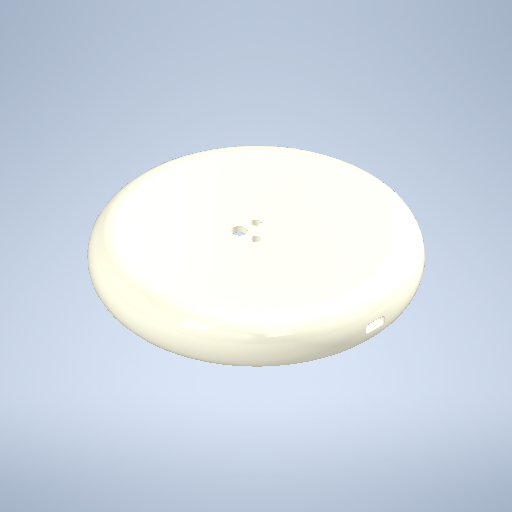
# Autodesk Inventor part: Base
Saved by Autodesk Inventor 2025.3 (Build 293356000, 356)
## iProperties
Created: 2026-01-15
Part Number: Base
Material: Acetal Resin, White
Document SubType Name: Modeling
Designer: Balint
Density: 1.425 g/cm^3
Appearance: Smooth - White
Mass: 112.917 g
Surface Area: 362.078 cm^2
Volume: 79.2398 cm^3
Author: Balint
Autodesk Inventor part; units mm, degrees
ref_plane "XZ Plane" through (0, 0, 0) normal (0, 1, 0) x (-1, 0, 0)
ref_plane "XY Plane" through (0, 0, 0) normal (0, 0, 1) x (1, 0, 0)
sketch "Sketch1" plane through (0, 0, 0) normal (0, 0, 1) x (1, 0, 0)
  line L0 (0, 0) -> (0, 22)
  line L1 (60, 5) -> (60, 5)
  line L2 (48.75, 19) -> (3, 19)
  line L3 (3, 19) -> (0, 19)
  line L4 (46.25, 0) -> (46.25, 2)
  line L5 (46.25, 2) -> (46.25, 3)
  line L6 (46.25, 3) -> (36.25, 3)
  line L7 (36.25, 3) -> (36.25, 6)
  line L8 (36.25, 6) -> (48.75, 6)
  line L9 (60, 11) -> (60, 11)
  line L10 (46.25, 0) -> (49, 0)
  line L11 (0, 22) -> (49, 22)
  arc A0 (60, 11) -> (49, 22) centre (49, 11) ccw
  arc A1 (49, 0) -> (60, 11) centre (49, 11) ccw
  line L12 (48.75, 6) -> (49.75, 6)
  line L13 (50.75, 7) -> (50.75, 18)
  line L14 (48.75, 19) -> (49.75, 19)
  arc A2 (50.75, 18) -> (49.75, 19) centre (49.75, 18) ccw
  arc A3 (49.75, 6) -> (50.75, 7) centre (49.75, 7) ccw
  point P0 (60, 22)
  point P1 (50.75, 6)
  dimension "d0" = 22
  dimension "d1" = 60
  dimension "d6" = 1
  dimension "d7" = 10
  dimension "d8" = 3
  dimension "d47" = 11
  dimension "d48" = 2
  dimension "d49" = 1
  constraints: 30 end point, 8 point on circle, 8 tangent, 6 perpendicular, 4 centre point, 3 horizontal, 3 point on line, 2 equal radius, 2 vertical
  measures "d0" distance of L0.start L0.end
  measures "d1" distance of L0.end point (60, 22)
  measures "d6" distance of L4.end L5.end
  measures "d7" distance of L5.end L6.end
  measures "d8" distance of L6.end L7.end
  measures "d47" radius of A0
  measures "d48" distance of L8.end point (50.75, 6)
  measures "d49" radius of A2
revolve "Revolution1" add sketch "Sketch1" angle 360 about axis through (0, 0, 0) along (0, 1, 0)
sketch "Sketch2" plane through (0, 3, 0) normal (0, -1, 0) x (1, 0, 0)
  circle A0 centre (0, 0) radius 36.25 projected
  circle A1 centre (0, 41.25) radius 1.9
  circle A2 centre (0, 0) radius 46.25 projected
  line L0 (0, 46.25) -> (0, 41.25)
  dimension "d11" = 3.8
  dimension "d38" = 5
  dimension "d39" = 0
  constraints: 2 end point, 1 centre point, 1 vertical, 1 vertical alignment, 1 other
  measures "d11" diameter of A1
  measures "d38" distance of L0.start L0.end
  measures "d39" distance of L0.end A1.centre
extrude "Extrusion1" cut sketch "Sketch2" against normal blind 4 contours A1
fillet "Fillet1" radius 0.5 3 edges at (-46.25, 0, 0) (-36.25, 3, 0) (-36.25, 6, 0)
pattern_circular "Circular Pattern1" count 4 over 360 about axis through (0, -10, 0) along (0, 1, 0) of "Extrusion1"
sketch "Sketch3" plane through (0, 19, 0) normal (0, -1, 0) x (1, 0, 0)
  circle A0 centre (0, 0) radius 12.5
  circle A1 centre (-4.2426, 4.2426) radius 3
  circle A2 centre (3.5355, 3.5355) radius 1.9
  circle A3 centre (-3.5355, -3.5355) radius 1.9
  circle A4 centre (-4.2426, 4.2426) radius 3
  circle A5 centre (3.5355, 3.5355) radius 1.9
  circle A6 centre (-3.5355, -3.5355) radius 1.9
  point P0 (0, 0)
  constraints: 7 centre point, 4 coincident, 3 concentric
extrude "Extrusion2" cut sketch "Sketch3" against normal blind 10 contours A1 | A2 | A3
fillet "Fillet2" radius 0.5 3 edges at (-5.4355, 19, -3.5355) (1.6355, 19, 3.5355) (-7.2426, 19, 4.2426)
ref_plane "Work Plane2" through (50, 0, 0) normal (1, 0, 0) x (0, 1, 0)
sketch "Sketch5" plane through (50, 0, 0) normal (1, 0, 0) x (0, 1, 0)
  line L0 (0, 0) -> (11, 0)
  line L1 (10.5, -4.4) -> (11.5, -4.4)
  line L2 (12.5, -3.4) -> (12.5, 3.4)
  line L3 (11.5, 4.4) -> (10.5, 4.4)
  line L4 (9.5, 3.4) -> (9.5, -3.4)
  line L5 (9.5, -4.4) -> (12.5, 4.4) construction
  line L6 (12.5, -4.4) -> (9.5, 4.4) construction
  arc A0 (12.5, 3.4) -> (11.5, 4.4) centre (11.5, 3.4) ccw
  arc A1 (10.5, 4.4) -> (9.5, 3.4) centre (10.5, 3.4) ccw
  arc A2 (11.5, -4.4) -> (12.5, -3.4) centre (11.5, -3.4) ccw
  arc A3 (9.5, -3.4) -> (10.5, -4.4) centre (10.5, -3.4) ccw
  dimension "d31" = 11
  dimension "d32" = 3
  dimension "d33" = 8.8
  dimension "d34" = 1
  constraints: 14 end point, 8 point on circle, 8 point on line, 8 tangent, 4 centre point, 3 equal radius, 2 horizontal, 2 midpoint, 2 parallel, 1 perpendicular
  measures "d31" distance of L0.start L0.end
  measures "d32" distance of L6.end L5.end
  measures "d33" distance of L5.end L6.start
  measures "d34" radius of A0
extrude "Extrusion4" cut sketch "Sketch5" along normal mid plane 27.25
fillet "Fillet6" radius 0.5 6 edges at (59.8356, 11.2501, 4.4) (59.7927, 12.2066, 4.1077) (59.8731, 12.5, 1.7007) (59.8731, 12.5, -1.7007) (59.7927, 12.2066, -4.1076) (59.8356, 11.2501, -4.4)
body "Solid1"
